Autodesk Fusion 360 part; units mm, degrees
(part 4 of 14)
  line L1260 (69.7278, -120.65) -> (64.2286, -111.125)
  line L1261 (64.2286, -130.175) -> (69.7278, -120.65)
  line L1262 (83.476, -100.0125) -> (72.4775, -100.0125)
  line L1263 (72.4775, -100.0125) -> (66.9782, -109.5375)
  line L1264 (66.9782, -109.5375) -> (72.4775, -119.0625)
  line L1265 (72.4775, -119.0625) -> (83.476, -119.0625)
  line L1266 (88.9753, -109.5375) -> (83.476, -100.0125)
  line L1267 (83.476, -119.0625) -> (88.9753, -109.5375)
  line L1268 (102.7234, -88.9) -> (91.7249, -88.9)
  line L1269 (91.7249, -88.9) -> (86.2256, -98.425)
  line L1270 (86.2256, -98.425) -> (91.7249, -107.95)
  line L1271 (91.7249, -107.95) -> (102.7234, -107.95)
  line L1272 (108.2227, -98.425) -> (102.7234, -88.9)
  line L1273 (102.7234, -107.95) -> (108.2227, -98.425)
  line L1274 (121.9708, -77.7875) -> (110.9723, -77.7875)
  line L1275 (110.9723, -77.7875) -> (105.473, -87.3125)
  line L1276 (105.473, -87.3125) -> (110.9723, -96.8375)
  line L1277 (110.9723, -96.8375) -> (121.9708, -96.8375)
  line L1278 (127.4701, -87.3125) -> (121.9708, -77.7875)
  line L1279 (121.9708, -96.8375) -> (127.4701, -87.3125)
  line L1280 (141.2182, -66.675) -> (130.2197, -66.675)
  line L1281 (130.2197, -66.675) -> (124.7205, -76.2)
  line L1282 (124.7205, -76.2) -> (130.2197, -85.725)
  line L1283 (130.2197, -85.725) -> (141.2182, -85.725)
  line L1284 (146.7175, -76.2) -> (141.2182, -66.675)
  line L1285 (141.2182, -85.725) -> (146.7175, -76.2)
  line L1286 (160.4657, -55.5625) -> (149.4671, -55.5625)
  line L1287 (149.4671, -55.5625) -> (143.9679, -65.0875)
  line L1288 (143.9679, -65.0875) -> (149.4671, -74.6125)
  line L1289 (149.4671, -74.6125) -> (160.4657, -74.6125)
  line L1290 (165.9649, -65.0875) -> (160.4657, -55.5625)
  line L1291 (160.4657, -74.6125) -> (165.9649, -65.0875)
  line L1292 (179.7131, -44.45) -> (168.7145, -44.45)
  line L1293 (168.7145, -44.45) -> (163.2153, -53.975)
  line L1294 (163.2153, -53.975) -> (168.7145, -63.5)
  line L1295 (168.7145, -63.5) -> (179.7131, -63.5)
  line L1296 (185.2123, -53.975) -> (179.7131, -44.45)
  line L1297 (179.7131, -63.5) -> (185.2123, -53.975)
  line L1298 (198.9605, -33.3375) -> (187.962, -33.3375)
  line L1299 (187.962, -33.3375) -> (182.4627, -42.8625)
  line L1300 (182.4627, -42.8625) -> (187.962, -52.3875)
  line L1301 (187.962, -52.3875) -> (198.9605, -52.3875)
  line L1302 (204.4597, -42.8625) -> (198.9605, -33.3375)
  line L1303 (198.9605, -52.3875) -> (204.4597, -42.8625)
  line L1304 (218.2079, -22.225) -> (207.2094, -22.225)
  line L1305 (207.2094, -22.225) -> (201.7101, -31.75)
  line L1306 (201.7101, -31.75) -> (207.2094, -41.275)
  line L1307 (207.2094, -41.275) -> (218.2079, -41.275)
  line L1308 (223.7072, -31.75) -> (218.2079, -22.225)
  line L1309 (218.2079, -41.275) -> (223.7072, -31.75)
  line L1310 (237.4553, -11.1125) -> (226.4568, -11.1125)
  line L1311 (226.4568, -11.1125) -> (220.9575, -20.6375)
  line L1312 (220.9575, -20.6375) -> (226.4568, -30.1625)
  line L1313 (226.4568, -30.1625) -> (237.4553, -30.1625)
  line L1314 (242.9546, -20.6375) -> (237.4553, -11.1125)
  line L1315 (237.4553, -30.1625) -> (242.9546, -20.6375)
  line L1316 (256.7027, 0) -> (245.7042, 0)
  line L1317 (245.7042, 0) -> (240.2049, -9.525)
  line L1318 (240.2049, -9.525) -> (245.7042, -19.05)
  line L1319 (245.7042, -19.05) -> (256.7027, -19.05)
  line L1320 (262.202, -9.525) -> (256.7027, 0)
  line L1321 (256.7027, -19.05) -> (262.202, -9.525)
  line L1322 (275.9501, 11.1125) -> (264.9516, 11.1125)
  line L1323 (264.9516, 11.1125) -> (259.4524, 1.5875)
  line L1324 (259.4524, 1.5875) -> (264.9516, -7.9375)
  line L1325 (264.9516, -7.9375) -> (275.9501, -7.9375)
  line L1326 (281.4494, 1.5875) -> (275.9501, 11.1125)
  line L1327 (275.9501, -7.9375) -> (281.4494, 1.5875)
  line L1328 (295.1976, 22.225) -> (284.199, 22.225)
  line L1329 (284.199, 22.225) -> (278.6998, 12.7)
  line L1330 (278.6998, 12.7) -> (284.199, 3.175)
  line L1331 (284.199, 3.175) -> (295.1976, 3.175)
  line L1332 (300.6968, 12.7) -> (295.1976, 22.225)
  line L1333 (295.1976, 3.175) -> (300.6968, 12.7)
  line L1334 (314.445, 33.3375) -> (303.4464, 33.3375)
  line L1335 (303.4464, 33.3375) -> (297.9472, 23.8125)
  line L1336 (297.9472, 23.8125) -> (303.4464, 14.2875)
  line L1337 (303.4464, 14.2875) -> (314.445, 14.2875)
  line L1338 (319.9442, 23.8125) -> (314.445, 33.3375)
  line L1339 (314.445, 14.2875) -> (319.9442, 23.8125)
  line L1340 (333.6924, 44.45) -> (322.6939, 44.45)
  line L1341 (322.6939, 44.45) -> (317.1946, 34.925)
  line L1342 (317.1946, 34.925) -> (322.6939, 25.4)
  line L1343 (322.6939, 25.4) -> (333.6924, 25.4)
  line L1344 (339.1916, 34.925) -> (333.6924, 44.45)
  line L1345 (333.6924, 25.4) -> (339.1916, 34.925)
  line L1346 (352.9398, 55.5625) -> (341.9413, 55.5625)
  line L1347 (341.9413, 55.5625) -> (336.442, 46.0375)
  line L1348 (336.442, 46.0375) -> (341.9413, 36.5125)
  line L1349 (341.9413, 36.5125) -> (352.9398, 36.5125)
  line L1350 (358.4391, 46.0375) -> (352.9398, 55.5625)
  line L1351 (352.9398, 36.5125) -> (358.4391, 46.0375)
  line L1352 (372.1872, 66.675) -> (361.1887, 66.675)
  line L1353 (361.1887, 66.675) -> (355.6894, 57.15)
  line L1354 (355.6894, 57.15) -> (361.1887, 47.625)
  line L1355 (361.1887, 47.625) -> (372.1872, 47.625)
  line L1356 (377.6865, 57.15) -> (372.1872, 66.675)
  line L1357 (372.1872, 47.625) -> (377.6865, 57.15)
  line L1358 (391.4346, 77.7875) -> (380.4361, 77.7875)
  line L1359 (380.4361, 77.7875) -> (374.9368, 68.2625)
  line L1360 (374.9368, 68.2625) -> (380.4361, 58.7375)
  line L1361 (380.4361, 58.7375) -> (391.4346, 58.7375)
  line L1362 (396.9339, 68.2625) -> (391.4346, 77.7875)
  line L1363 (391.4346, 58.7375) -> (396.9339, 68.2625)
  line L1364 (410.682, 88.9) -> (399.6835, 88.9)
  line L1365 (399.6835, 88.9) -> (394.1843, 79.375)
  line L1366 (394.1843, 79.375) -> (399.6835, 69.85)
  line L1367 (399.6835, 69.85) -> (410.682, 69.85)
  line L1368 (416.1813, 79.375) -> (410.682, 88.9)
  line L1369 (410.682, 69.85) -> (416.1813, 79.375)
  line L1370 (429.9295, 100.0125) -> (418.9309, 100.0125)
  line L1371 (418.9309, 100.0125) -> (413.4317, 90.4875)
  line L1372 (413.4317, 90.4875) -> (418.9309, 80.9625)
  line L1373 (418.9309, 80.9625) -> (429.9295, 80.9625)
  line L1374 (435.4287, 90.4875) -> (429.9295, 100.0125)
  line L1375 (429.9295, 80.9625) -> (435.4287, 90.4875)
  line L1376 (449.1769, 111.125) -> (438.1783, 111.125)
  line L1377 (438.1783, 111.125) -> (432.6791, 101.6)
  line L1378 (432.6791, 101.6) -> (438.1783, 92.075)
  line L1379 (438.1783, 92.075) -> (449.1769, 92.075)
  line L1380 (454.6761, 101.6) -> (449.1769, 111.125)
  line L1381 (449.1769, 92.075) -> (454.6761, 101.6)
  line L1382 (468.4243, 122.2375) -> (457.4258, 122.2375)
  line L1383 (457.4258, 122.2375) -> (451.9265, 112.7125)
  line L1384 (451.9265, 112.7125) -> (457.4258, 103.1875)
  line L1385 (457.4258, 103.1875) -> (468.4243, 103.1875)
  line L1386 (473.9235, 112.7125) -> (468.4243, 122.2375)
  line L1387 (468.4243, 103.1875) -> (473.9235, 112.7125)
  line L1388 (487.6717, 133.35) -> (476.6732, 133.35)
  line L1389 (476.6732, 133.35) -> (471.1739, 123.825)
  line L1390 (471.1739, 123.825) -> (476.6732, 114.3)
  line L1391 (476.6732, 114.3) -> (487.6717, 114.3)
  line L1392 (493.171, 123.825) -> (487.6717, 133.35)
  line L1393 (487.6717, 114.3) -> (493.171, 123.825)
  line L1394 (506.9191, 144.4625) -> (495.9206, 144.4625)
  line L1395 (495.9206, 144.4625) -> (490.4213, 134.9375)
  line L1396 (490.4213, 134.9375) -> (495.9206, 125.4125)
  line L1397 (495.9206, 125.4125) -> (506.9191, 125.4125)
  line L1398 (512.4184, 134.9375) -> (506.9191, 144.4625)
  line L1399 (506.9191, 125.4125) -> (512.4184, 134.9375)
  line L1400 (526.1665, 155.575) -> (515.168, 155.575)
  line L1401 (515.168, 155.575) -> (509.6687, 146.05)
  line L1402 (509.6687, 146.05) -> (515.168, 136.525)
  line L1403 (515.168, 136.525) -> (526.1665, 136.525)
  line L1404 (531.6658, 146.05) -> (526.1665, 155.575)
  line L1405 (526.1665, 136.525) -> (531.6658, 146.05)
  line L1406 (545.4139, 166.6875) -> (534.4154, 166.6875)
  line L1407 (534.4154, 166.6875) -> (528.9162, 157.1625)
  line L1408 (528.9162, 157.1625) -> (534.4154, 147.6375)
  line L1409 (534.4154, 147.6375) -> (545.4139, 147.6375)
  line L1410 (550.9132, 157.1625) -> (545.4139, 166.6875)
  line L1411 (545.4139, 147.6375) -> (550.9132, 157.1625)
  line L1412 (564.6614, 177.8) -> (553.6628, 177.8)
  line L1413 (553.6628, 177.8) -> (548.1636, 168.275)
  line L1414 (548.1636, 168.275) -> (553.6628, 158.75)
  line L1415 (553.6628, 158.75) -> (564.6614, 158.75)
  line L1416 (570.1606, 168.275) -> (564.6614, 177.8)
  line L1417 (564.6614, 158.75) -> (570.1606, 168.275)
  line L1418 (583.9088, 188.9125) -> (572.9102, 188.9125)
  line L1419 (572.9102, 188.9125) -> (567.411, 179.3875)
  line L1420 (567.411, 179.3875) -> (572.9102, 169.8625)
  line L1421 (572.9102, 169.8625) -> (583.9088, 169.8625)
  line L1422 (589.408, 179.3875) -> (583.9088, 188.9125)
  line L1423 (583.9088, 169.8625) -> (589.408, 179.3875)
  line L1424 (603.1562, 200.025) -> (592.1577, 200.025)
  line L1425 (592.1577, 200.025) -> (586.6584, 190.5)
  line L1426 (586.6584, 190.5) -> (592.1577, 180.975)
  line L1427 (592.1577, 180.975) -> (603.1562, 180.975)
  line L1428 (608.6554, 190.5) -> (603.1562, 200.025)
  line L1429 (603.1562, 180.975) -> (608.6554, 190.5)
  line L1430 (622.4036, 211.1375) -> (611.4051, 211.1375)
  line L1431 (611.4051, 211.1375) -> (605.9058, 201.6125)
  line L1432 (605.9058, 201.6125) -> (611.4051, 192.0875)
  line L1433 (611.4051, 192.0875) -> (622.4036, 192.0875)
  line L1434 (627.9029, 201.6125) -> (622.4036, 211.1375)
  line L1435 (622.4036, 192.0875) -> (627.9029, 201.6125)
  line L1436 (641.651, 222.25) -> (630.6525, 222.25)
  line L1437 (630.6525, 222.25) -> (625.1532, 212.725)
  line L1438 (625.1532, 212.725) -> (630.6525, 203.2)
  line L1439 (630.6525, 203.2) -> (641.651, 203.2)
  line L1440 (647.1503, 212.725) -> (641.651, 222.25)
  line L1441 (641.651, 203.2) -> (647.1503, 212.725)
  line L1442 (660.8984, 233.3625) -> (649.8999, 233.3625)
  line L1443 (649.8999, 233.3625) -> (644.4006, 223.8375)
  line L1444 (644.4006, 223.8375) -> (649.8999, 214.3125)
  line L1445 (649.8999, 214.3125) -> (660.8984, 214.3125)
  line L1446 (666.3977, 223.8375) -> (660.8984, 233.3625)
  line L1447 (660.8984, 214.3125) -> (666.3977, 223.8375)
  line L1448 (680.1458, 244.475) -> (669.1473, 244.475)
  line L1449 (669.1473, 244.475) -> (663.6481, 234.95)
  line L1450 (663.6481, 234.95) -> (669.1473, 225.425)
  line L1451 (669.1473, 225.425) -> (680.1458, 225.425)
  line L1452 (685.6451, 234.95) -> (680.1458, 244.475)
  line L1453 (680.1458, 225.425) -> (685.6451, 234.95)
  line L1454 (699.3933, 255.5875) -> (688.3947, 255.5875)
  line L1455 (688.3947, 255.5875) -> (682.8955, 246.0625)
  line L1456 (682.8955, 246.0625) -> (688.3947, 236.5375)
  line L1457 (688.3947, 236.5375) -> (699.3933, 236.5375)
  line L1458 (704.8925, 246.0625) -> (699.3933, 255.5875)
  line L1459 (699.3933, 236.5375) -> (704.8925, 246.0625)
  line L1460 (-455.4516, -388.9375) -> (-466.4501, -388.9375)
  line L1461 (-466.4501, -388.9375) -> (-471.9494, -398.4625)
  line L1462 (-471.9494, -398.4625) -> (-466.4501, -407.9875)
  line L1463 (-466.4501, -407.9875) -> (-455.4516, -407.9875)
  line L1464 (-449.9524, -398.4625) -> (-455.4516, -388.9375)
  line L1465 (-455.4516, -407.9875) -> (-449.9524, -398.4625)
  line L1466 (-436.2042, -377.825) -> (-447.2027, -377.825)
  line L1467 (-447.2027, -377.825) -> (-452.702, -387.35)
  line L1468 (-452.702, -387.35) -> (-447.2027, -396.875)
  line L1469 (-447.2027, -396.875) -> (-436.2042, -396.875)
  line L1470 (-430.7049, -387.35) -> (-436.2042, -377.825)
  line L1471 (-436.2042, -396.875) -> (-430.7049, -387.35)
  line L1472 (-416.9568, -366.7125) -> (-427.9553, -366.7125)
  line L1473 (-427.9553, -366.7125) -> (-433.4546, -376.2375)
  line L1474 (-433.4546, -376.2375) -> (-427.9553, -385.7625)
  line L1475 (-427.9553, -385.7625) -> (-416.9568, -385.7625)
  line L1476 (-411.4575, -376.2375) -> (-416.9568, -366.7125)
  line L1477 (-416.9568, -385.7625) -> (-411.4575, -376.2375)
  line L1478 (-397.7094, -355.6) -> (-408.7079, -355.6)
  line L1479 (-408.7079, -355.6) -> (-414.2072, -365.125)
  line L1480 (-414.2072, -365.125) -> (-408.7079, -374.65)
  line L1481 (-408.7079, -374.65) -> (-397.7094, -374.65)
  line L1482 (-392.2101, -365.125) -> (-397.7094, -355.6)
  line L1483 (-397.7094, -374.65) -> (-392.2101, -365.125)
  line L1484 (-378.462, -344.4875) -> (-389.4605, -344.4875)
  line L1485 (-389.4605, -344.4875) -> (-394.9597, -354.0125)
  line L1486 (-394.9597, -354.0125) -> (-389.4605, -363.5375)
  line L1487 (-389.4605, -363.5375) -> (-378.462, -363.5375)
  line L1488 (-372.9627, -354.0125) -> (-378.462, -344.4875)
  line L1489 (-378.462, -363.5375) -> (-372.9627, -354.0125)
  line L1490 (-359.2145, -333.375) -> (-370.2131, -333.375)
  line L1491 (-370.2131, -333.375) -> (-375.7123, -342.9)
  line L1492 (-375.7123, -342.9) -> (-370.2131, -352.425)
  line L1493 (-370.2131, -352.425) -> (-359.2145, -352.425)
  line L1494 (-353.7153, -342.9) -> (-359.2145, -333.375)
  line L1495 (-359.2145, -352.425) -> (-353.7153, -342.9)
  line L1496 (-339.9671, -322.2625) -> (-350.9657, -322.2625)
  line L1497 (-350.9657, -322.2625) -> (-356.4649, -331.7875)
  line L1498 (-356.4649, -331.7875) -> (-350.9657, -341.3125)
  line L1499 (-350.9657, -341.3125) -> (-339.9671, -341.3125)
  line L1500 (-334.4679, -331.7875) -> (-339.9671, -322.2625)
  line L1501 (-339.9671, -341.3125) -> (-334.4679, -331.7875)
  line L1502 (-320.7197, -311.15) -> (-331.7182, -311.15)
  line L1503 (-331.7182, -311.15) -> (-337.2175, -320.675)
  line L1504 (-337.2175, -320.675) -> (-331.7182, -330.2)
  line L1505 (-331.7182, -330.2) -> (-320.7197, -330.2)
  line L1506 (-315.2205, -320.675) -> (-320.7197, -311.15)
  line L1507 (-320.7197, -330.2) -> (-315.2205, -320.675)
  line L1508 (-301.4723, -300.0375) -> (-312.4708, -300.0375)
  line L1509 (-312.4708, -300.0375) -> (-317.9701, -309.5625)
  line L1510 (-317.9701, -309.5625) -> (-312.4708, -319.0875)
  line L1511 (-312.4708, -319.0875) -> (-301.4723, -319.0875)
  line L1512 (-295.973, -309.5625) -> (-301.4723, -300.0375)
  line L1513 (-301.4723, -319.0875) -> (-295.973, -309.5625)
  line L1514 (-282.2249, -288.925) -> (-293.2234, -288.925)
  line L1515 (-293.2234, -288.925) -> (-298.7227, -298.45)
  line L1516 (-298.7227, -298.45) -> (-293.2234, -307.975)
  line L1517 (-293.2234, -307.975) -> (-282.2249, -307.975)
  line L1518 (-276.7256, -298.45) -> (-282.2249, -288.925)
  line L1519 (-282.2249, -307.975) -> (-276.7256, -298.45)
  line L1520 (-262.9775, -277.8125) -> (-273.976, -277.8125)
  line L1521 (-273.976, -277.8125) -> (-279.4753, -287.3375)
  line L1522 (-279.4753, -287.3375) -> (-273.976, -296.8625)
  line L1523 (-273.976, -296.8625) -> (-262.9775, -296.8625)
  line L1524 (-257.4782, -287.3375) -> (-262.9775, -277.8125)
  line L1525 (-262.9775, -296.8625) -> (-257.4782, -287.3375)
  line L1526 (-243.7301, -266.7) -> (-254.7286, -266.7)
  line L1527 (-254.7286, -266.7) -> (-260.2278, -276.225)
  line L1528 (-260.2278, -276.225) -> (-254.7286, -285.75)
  line L1529 (-254.7286, -285.75) -> (-243.7301, -285.75)
  line L1530 (-238.2308, -276.225) -> (-243.7301, -266.7)
  line L1531 (-243.7301, -285.75) -> (-238.2308, -276.225)
  line L1532 (-224.4826, -255.5875) -> (-235.4812, -255.5875)
  line L1533 (-235.4812, -255.5875) -> (-240.9804, -265.1125)
  line L1534 (-240.9804, -265.1125) -> (-235.4812, -274.6375)
  line L1535 (-235.4812, -274.6375) -> (-224.4826, -274.6375)
  line L1536 (-218.9834, -265.1125) -> (-224.4826, -255.5875)
  line L1537 (-224.4826, -274.6375) -> (-218.9834, -265.1125)
  line L1538 (-205.2352, -244.475) -> (-216.2337, -244.475)
  line L1539 (-216.2337, -244.475) -> (-221.733, -254)
  line L1540 (-221.733, -254) -> (-216.2337, -263.525)
  line L1541 (-216.2337, -263.525) -> (-205.2352, -263.525)
  line L1542 (-199.736, -254) -> (-205.2352, -244.475)
  line L1543 (-205.2352, -263.525) -> (-199.736, -254)
  line L1544 (-185.9878, -233.3625) -> (-196.9863, -233.3625)
  line L1545 (-196.9863, -233.3625) -> (-202.4856, -242.8875)
  line L1546 (-202.4856, -242.8875) -> (-196.9863, -252.4125)
  line L1547 (-196.9863, -252.4125) -> (-185.9878, -252.4125)
  line L1548 (-180.4886, -242.8875) -> (-185.9878, -233.3625)
  line L1549 (-185.9878, -252.4125) -> (-180.4886, -242.8875)
  line L1550 (-166.7404, -222.25) -> (-177.7389, -222.25)
  line L1551 (-177.7389, -222.25) -> (-183.2382, -231.775)
  line L1552 (-183.2382, -231.775) -> (-177.7389, -241.3)
  line L1553 (-177.7389, -241.3) -> (-166.7404, -241.3)
  line L1554 (-161.2411, -231.775) -> (-166.7404, -222.25)
  line L1555 (-166.7404, -241.3) -> (-161.2411, -231.775)
  line L1556 (-147.493, -211.1375) -> (-158.4915, -211.1375)
  line L1557 (-158.4915, -211.1375) -> (-163.9908, -220.6625)
  line L1558 (-163.9908, -220.6625) -> (-158.4915, -230.1875)
  line L1559 (-158.4915, -230.1875) -> (-147.493, -230.1875)
  line L1560 (-141.9937, -220.6625) -> (-147.493, -211.1375)
  line L1561 (-147.493, -230.1875) -> (-141.9937, -220.6625)
  line L1562 (-128.2456, -200.025) -> (-139.2441, -200.025)
  line L1563 (-139.2441, -200.025) -> (-144.7434, -209.55)
  line L1564 (-144.7434, -209.55) -> (-139.2441, -219.075)
  line L1565 (-139.2441, -219.075) -> (-128.2456, -219.075)
  line L1566 (-122.7463, -209.55) -> (-128.2456, -200.025)
  line L1567 (-128.2456, -219.075) -> (-122.7463, -209.55)
  line L1568 (-108.9982, -188.9125) -> (-119.9967, -188.9125)
  line L1569 (-119.9967, -188.9125) -> (-125.4959, -198.4375)
  line L1570 (-125.4959, -198.4375) -> (-119.9967, -207.9625)
  line L1571 (-119.9967, -207.9625) -> (-108.9982, -207.9625)
  line L1572 (-103.4989, -198.4375) -> (-108.9982, -188.9125)
  line L1573 (-108.9982, -207.9625) -> (-103.4989, -198.4375)
  line L1574 (-89.7507, -177.8) -> (-100.7493, -177.8)
  line L1575 (-100.7493, -177.8) -> (-106.2485, -187.325)
  line L1576 (-106.2485, -187.325) -> (-100.7493, -196.85)
  line L1577 (-100.7493, -196.85) -> (-89.7507, -196.85)
  line L1578 (-84.2515, -187.325) -> (-89.7507, -177.8)
  line L1579 (-89.7507, -196.85) -> (-84.2515, -187.325)
  line L1580 (-70.5033, -166.6875) -> (-81.5018, -166.6875)
  line L1581 (-81.5018, -166.6875) -> (-87.0011, -176.2125)
  line L1582 (-87.0011, -176.2125) -> (-81.5018, -185.7375)
  line L1583 (-81.5018, -185.7375) -> (-70.5033, -185.7375)
  line L1584 (-65.0041, -176.2125) -> (-70.5033, -166.6875)
  line L1585 (-70.5033, -185.7375) -> (-65.0041, -176.2125)
  line L1586 (-51.2559, -155.575) -> (-62.2544, -155.575)
  line L1587 (-62.2544, -155.575) -> (-67.7537, -165.1)
  line L1588 (-67.7537, -165.1) -> (-62.2544, -174.625)
  line L1589 (-62.2544, -174.625) -> (-51.2559, -174.625)
  line L1590 (-45.7566, -165.1) -> (-51.2559, -155.575)
  line L1591 (-51.2559, -174.625) -> (-45.7566, -165.1)
  line L1592 (-32.0085, -144.4625) -> (-43.007, -144.4625)
  line L1593 (-43.007, -144.4625) -> (-48.5063, -153.9875)
  line L1594 (-48.5063, -153.9875) -> (-43.007, -163.5125)
  line L1595 (-43.007, -163.5125) -> (-32.0085, -163.5125)
  line L1596 (-26.5092, -153.9875) -> (-32.0085, -144.4625)
  line L1597 (-32.0085, -163.5125) -> (-26.5092, -153.9875)
  line L1598 (-12.7611, -133.35) -> (-23.7596, -133.35)
  line L1599 (-23.7596, -133.35) -> (-29.2589, -142.875)
  line L1600 (-29.2589, -142.875) -> (-23.7596, -152.4)
  line L1601 (-23.7596, -152.4) -> (-12.7611, -152.4)
  line L1602 (-7.2618, -142.875) -> (-12.7611, -133.35)
  line L1603 (-12.7611, -152.4) -> (-7.2618, -142.875)
  line L1604 (6.4863, -122.2375) -> (-4.5122, -122.2375)
  line L1605 (-4.5122, -122.2375) -> (-10.0114, -131.7625)
  line L1606 (-10.0114, -131.7625) -> (-4.5122, -141.2875)
  line L1607 (-4.5122, -141.2875) -> (6.4863, -141.2875)
  line L1608 (11.9856, -131.7625) -> (6.4863, -122.2375)
  line L1609 (6.4863, -141.2875) -> (11.9856, -131.7625)
  line L1610 (25.7337, -111.125) -> (14.7352, -111.125)
  line L1611 (14.7352, -111.125) -> (9.236, -120.65)
  line L1612 (9.236, -120.65) -> (14.7352, -130.175)
  line L1613 (14.7352, -130.175) -> (25.7337, -130.175)
  line L1614 (31.233, -120.65) -> (25.7337, -111.125)
  line L1615 (25.7337, -130.175) -> (31.233, -120.65)
  line L1616 (44.9812, -100.0125) -> (33.9826, -100.0125)
  line L1617 (33.9826, -100.0125) -> (28.4834, -109.5375)
  line L1618 (28.4834, -109.5375) -> (33.9826, -119.0625)
  line L1619 (33.9826, -119.0625) -> (44.9812, -119.0625)
  line L1620 (50.4804, -109.5375) -> (44.9812, -100.0125)
  line L1621 (44.9812, -119.0625) -> (50.4804, -109.5375)
  line L1622 (64.2286, -88.9) -> (53.2301, -88.9)
  line L1623 (53.2301, -88.9) -> (47.7308, -98.425)
  line L1624 (47.7308, -98.425) -> (53.2301, -107.95)
  line L1625 (53.2301, -107.95) -> (64.2286, -107.95)
  line L1626 (69.7278, -98.425) -> (64.2286, -88.9)
  line L1627 (64.2286, -107.95) -> (69.7278, -98.425)
  line L1628 (83.476, -77.7875) -> (72.4775, -77.7875)
  line L1629 (72.4775, -77.7875) -> (66.9782, -87.3125)
  line L1630 (66.9782, -87.3125) -> (72.4775, -96.8375)
  line L1631 (72.4775, -96.8375) -> (83.476, -96.8375)
  line L1632 (88.9753, -87.3125) -> (83.476, -77.7875)
  line L1633 (83.476, -96.8375) -> (88.9753, -87.3125)
  line L1634 (102.7234, -66.675) -> (91.7249, -66.675)
  line L1635 (91.7249, -66.675) -> (86.2256, -76.2)
  line L1636 (86.2256, -76.2) -> (91.7249, -85.725)
  line L1637 (91.7249, -85.725) -> (102.7234, -85.725)
  line L1638 (108.2227, -76.2) -> (102.7234, -66.675)
  line L1639 (102.7234, -85.725) -> (108.2227, -76.2)
  line L1640 (121.9708, -55.5625) -> (110.9723, -55.5625)
  line L1641 (110.9723, -55.5625) -> (105.473, -65.0875)
  line L1642 (105.473, -65.0875) -> (110.9723, -74.6125)
  line L1643 (110.9723, -74.6125) -> (121.9708, -74.6125)
  line L1644 (127.4701, -65.0875) -> (121.9708, -55.5625)
  line L1645 (121.9708, -74.6125) -> (127.4701, -65.0875)
  line L1646 (141.2182, -44.45) -> (130.2197, -44.45)
  line L1647 (130.2197, -44.45) -> (124.7205, -53.975)
  line L1648 (124.7205, -53.975) -> (130.2197, -63.5)
  line L1649 (130.2197, -63.5) -> (141.2182, -63.5)
  line L1650 (146.7175, -53.975) -> (141.2182, -44.45)
  line L1651 (141.2182, -63.5) -> (146.7175, -53.975)
  line L1652 (160.4657, -33.3375) -> (149.4671, -33.3375)
  line L1653 (149.4671, -33.3375) -> (143.9679, -42.8625)
  line L1654 (143.9679, -42.8625) -> (149.4671, -52.3875)
  line L1655 (149.4671, -52.3875) -> (160.4657, -52.3875)
  line L1656 (165.9649, -42.8625) -> (160.4657, -33.3375)
  line L1657 (160.4657, -52.3875) -> (165.9649, -42.8625)
  line L1658 (179.7131, -22.225) -> (168.7145, -22.225)
  line L1659 (168.7145, -22.225) -> (163.2153, -31.75)
  line L1660 (163.2153, -31.75) -> (168.7145, -41.275)
  line L1661 (168.7145, -41.275) -> (179.7131, -41.275)
  line L1662 (185.2123, -31.75) -> (179.7131, -22.225)
  line L1663 (179.7131, -41.275) -> (185.2123, -31.75)
  line L1664 (198.9605, -11.1125) -> (187.962, -11.1125)
  line L1665 (187.962, -11.1125) -> (182.4627, -20.6375)
  line L1666 (182.4627, -20.6375) -> (187.962, -30.1625)
  line L1667 (187.962, -30.1625) -> (198.9605, -30.1625)
  line L1668 (204.4597, -20.6375) -> (198.9605, -11.1125)
  line L1669 (198.9605, -30.1625) -> (204.4597, -20.6375)
  line L1670 (218.2079, 0) -> (207.2094, 0)
  line L1671 (207.2094, 0) -> (201.7101, -9.525)
  line L1672 (201.7101, -9.525) -> (207.2094, -19.05)
  line L1673 (207.2094, -19.05) -> (218.2079, -19.05)
  line L1674 (223.7072, -9.525) -> (218.2079, 0)
  line L1675 (218.2079, -19.05) -> (223.7072, -9.525)
  line L1676 (237.4553, 11.1125) -> (226.4568, 11.1125)
  line L1677 (226.4568, 11.1125) -> (220.9575, 1.5875)
  line L1678 (220.9575, 1.5875) -> (226.4568, -7.9375)
  line L1679 (226.4568, -7.9375) -> (237.4553, -7.9375)
  line L1680 (242.9546, 1.5875) -> (237.4553, 11.1125)
  line L1681 (237.4553, -7.9375) -> (242.9546, 1.5875)
  line L1682 (256.7027, 22.225) -> (245.7042, 22.225)
  line L1683 (245.7042, 22.225) -> (240.2049, 12.7)
  line L1684 (240.2049, 12.7) -> (245.7042, 3.175)
  line L1685 (245.7042, 3.175) -> (256.7027, 3.175)
  line L1686 (262.202, 12.7) -> (256.7027, 22.225)
  line L1687 (256.7027, 3.175) -> (262.202, 12.7)
  line L1688 (275.9501, 33.3375) -> (264.9516, 33.3375)
  line L1689 (264.9516, 33.3375) -> (259.4524, 23.8125)
  line L1690 (259.4524, 23.8125) -> (264.9516, 14.2875)
  line L1691 (264.9516, 14.2875) -> (275.9501, 14.2875)
  line L1692 (281.4494, 23.8125) -> (275.9501, 33.3375)
  line L1693 (275.9501, 14.2875) -> (281.4494, 23.8125)
  line L1694 (295.1976, 44.45) -> (284.199, 44.45)
  line L1695 (284.199, 44.45) -> (278.6998, 34.925)
  line L1696 (278.6998, 34.925) -> (284.199, 25.4)
  line L1697 (284.199, 25.4) -> (295.1976, 25.4)
  line L1698 (300.6968, 34.925) -> (295.1976, 44.45)
  line L1699 (295.1976, 25.4) -> (300.6968, 34.925)
  line L1700 (314.445, 55.5625) -> (303.4464, 55.5625)
  line L1701 (303.4464, 55.5625) -> (297.9472, 46.0375)
  line L1702 (297.9472, 46.0375) -> (303.4464, 36.5125)
  line L1703 (303.4464, 36.5125) -> (314.445, 36.5125)
  line L1704 (319.9442, 46.0375) -> (314.445, 55.5625)
  line L1705 (314.445, 36.5125) -> (319.9442, 46.0375)
  line L1706 (333.6924, 66.675) -> (322.6939, 66.675)
  line L1707 (322.6939, 66.675) -> (317.1946, 57.15)
  line L1708 (317.1946, 57.15) -> (322.6939, 47.625)
  line L1709 (322.6939, 47.625) -> (333.6924, 47.625)
  line L1710 (339.1916, 57.15) -> (333.6924, 66.675)
  line L1711 (333.6924, 47.625) -> (339.1916, 57.15)
  line L1712 (352.9398, 77.7875) -> (341.9413, 77.7875)
  line L1713 (341.9413, 77.7875) -> (336.442, 68.2625)
  line L1714 (336.442, 68.2625) -> (341.9413, 58.7375)
  line L1715 (341.9413, 58.7375) -> (352.9398, 58.7375)
  line L1716 (358.4391, 68.2625) -> (352.9398, 77.7875)
  line L1717 (352.9398, 58.7375) -> (358.4391, 68.2625)
  line L1718 (372.1872, 88.9) -> (361.1887, 88.9)
  line L1719 (361.1887, 88.9) -> (355.6894, 79.375)
  line L1720 (355.6894, 79.375) -> (361.1887, 69.85)
  line L1721 (361.1887, 69.85) -> (372.1872, 69.85)
  line L1722 (377.6865, 79.375) -> (372.1872, 88.9)
  line L1723 (372.1872, 69.85) -> (377.6865, 79.375)
  line L1724 (391.4346, 100.0125) -> (380.4361, 100.0125)
  line L1725 (380.4361, 100.0125) -> (374.9368, 90.4875)
  line L1726 (374.9368, 90.4875) -> (380.4361, 80.9625)
  line L1727 (380.4361, 80.9625) -> (391.4346, 80.9625)
  line L1728 (396.9339, 90.4875) -> (391.4346, 100.0125)
  line L1729 (391.4346, 80.9625) -> (396.9339, 90.4875)
  line L1730 (410.682, 111.125) -> (399.6835, 111.125)
  line L1731 (399.6835, 111.125) -> (394.1843, 101.6)
  line L1732 (394.1843, 101.6) -> (399.6835, 92.075)
  line L1733 (399.6835, 92.075) -> (410.682, 92.075)
  line L1734 (416.1813, 101.6) -> (410.682, 111.125)
  line L1735 (410.682, 92.075) -> (416.1813, 101.6)
  line L1736 (429.9295, 122.2375) -> (418.9309, 122.2375)
  line L1737 (418.9309, 122.2375) -> (413.4317, 112.7125)
  line L1738 (413.4317, 112.7125) -> (418.9309, 103.1875)
  line L1739 (418.9309, 103.1875) -> (429.9295, 103.1875)
  line L1740 (435.4287, 112.7125) -> (429.9295, 122.2375)
  line L1741 (429.9295, 103.1875) -> (435.4287, 112.7125)
  line L1742 (449.1769, 133.35) -> (438.1783, 133.35)
  line L1743 (438.1783, 133.35) -> (432.6791, 123.825)
  line L1744 (432.6791, 123.825) -> (438.1783, 114.3)
  line L1745 (438.1783, 114.3) -> (449.1769, 114.3)
  line L1746 (454.6761, 123.825) -> (449.1769, 133.35)
  line L1747 (449.1769, 114.3) -> (454.6761, 123.825)
  line L1748 (468.4243, 144.4625) -> (457.4258, 144.4625)
  line L1749 (457.4258, 144.4625) -> (451.9265, 134.9375)
  line L1750 (451.9265, 134.9375) -> (457.4258, 125.4125)
  line L1751 (457.4258, 125.4125) -> (468.4243, 125.4125)
  line L1752 (473.9235, 134.9375) -> (468.4243, 144.4625)
  line L1753 (468.4243, 125.4125) -> (473.9235, 134.9375)
  line L1754 (487.6717, 155.575) -> (476.6732, 155.575)
  line L1755 (476.6732, 155.575) -> (471.1739, 146.05)
  line L1756 (471.1739, 146.05) -> (476.6732, 136.525)
  line L1757 (476.6732, 136.525) -> (487.6717, 136.525)
  line L1758 (493.171, 146.05) -> (487.6717, 155.575)
  line L1759 (487.6717, 136.525) -> (493.171, 146.05)
  line L1760 (506.9191, 166.6875) -> (495.9206, 166.6875)
  line L1761 (495.9206, 166.6875) -> (490.4213, 157.1625)
  line L1762 (490.4213, 157.1625) -> (495.9206, 147.6375)
  line L1763 (495.9206, 147.6375) -> (506.9191, 147.6375)
  line L1764 (512.4184, 157.1625) -> (506.9191, 166.6875)
  line L1765 (506.9191, 147.6375) -> (512.4184, 157.1625)
  line L1766 (526.1665, 177.8) -> (515.168, 177.8)
  line L1767 (515.168, 177.8) -> (509.6687, 168.275)
  line L1768 (509.6687, 168.275) -> (515.168, 158.75)
  line L1769 (515.168, 158.75) -> (526.1665, 158.75)
  line L1770 (531.6658, 168.275) -> (526.1665, 177.8)
  line L1771 (526.1665, 158.75) -> (531.6658, 168.275)
  line L1772 (545.4139, 188.9125) -> (534.4154, 188.9125)
  line L1773 (534.4154, 188.9125) -> (528.9162, 179.3875)
  line L1774 (528.9162, 179.3875) -> (534.4154, 169.8625)
  line L1775 (534.4154, 169.8625) -> (545.4139, 169.8625)
  line L1776 (550.9132, 179.3875) -> (545.4139, 188.9125)
  line L1777 (545.4139, 169.8625) -> (550.9132, 179.3875)
  line L1778 (564.6614, 200.025) -> (553.6628, 200.025)
  line L1779 (553.6628, 200.025) -> (548.1636, 190.5)
  line L1780 (548.1636, 190.5) -> (553.6628, 180.975)
  line L1781 (553.6628, 180.975) -> (564.6614, 180.975)
  line L1782 (570.1606, 190.5) -> (564.6614, 200.025)
  line L1783 (564.6614, 180.975) -> (570.1606, 190.5)
  line L1784 (583.9088, 211.1375) -> (572.9102, 211.1375)
  line L1785 (572.9102, 211.1375) -> (567.411, 201.6125)
  line L1786 (567.411, 201.6125) -> (572.9102, 192.0875)
  line L1787 (572.9102, 192.0875) -> (583.9088, 192.0875)
  line L1788 (589.408, 201.6125) -> (583.9088, 211.1375)
  line L1789 (583.9088, 192.0875) -> (589.408, 201.6125)
  line L1790 (603.1562, 222.25) -> (592.1577, 222.25)
  line L1791 (592.1577, 222.25) -> (586.6584, 212.725)
  line L1792 (586.6584, 212.725) -> (592.1577, 203.2)
  line L1793 (592.1577, 203.2) -> (603.1562, 203.2)
  line L1794 (608.6554, 212.725) -> (603.1562, 222.25)
  line L1795 (603.1562, 203.2) -> (608.6554, 212.725)
  line L1796 (622.4036, 233.3625) -> (611.4051, 233.3625)
  line L1797 (611.4051, 233.3625) -> (605.9058, 223.8375)
  line L1798 (605.9058, 223.8375) -> (611.4051, 214.3125)
  line L1799 (611.4051, 214.3125) -> (622.4036, 214.3125)
  line L1800 (627.9029, 223.8375) -> (622.4036, 233.3625)
  line L1801 (622.4036, 214.3125) -> (627.9029, 223.8375)
  line L1802 (641.651, 244.475) -> (630.6525, 244.475)
  line L1803 (630.6525, 244.475) -> (625.1532, 234.95)
  line L1804 (625.1532, 234.95) -> (630.6525, 225.425)
  line L1805 (630.6525, 225.425) -> (641.651, 225.425)
  line L1806 (647.1503, 234.95) -> (641.651, 244.475)
  line L1807 (641.651, 225.425) -> (647.1503, 234.95)
  line L1808 (660.8984, 255.5875) -> (649.8999, 255.5875)
  line L1809 (649.8999, 255.5875) -> (644.4006, 246.0625)
  line L1810 (644.4006, 246.0625) -> (649.8999, 236.5375)
  line L1811 (649.8999, 236.5375) -> (660.8984, 236.5375)
  line L1812 (666.3977, 246.0625) -> (660.8984, 255.5875)
  line L1813 (660.8984, 236.5375) -> (666.3977, 246.0625)
  line L1814 (680.1458, 266.7) -> (669.1473, 266.7)
  line L1815 (669.1473, 266.7) -> (663.6481, 257.175)
  line L1816 (663.6481, 257.175) -> (669.1473, 247.65)
  line L1817 (669.1473, 247.65) -> (680.1458, 247.65)
  line L1818 (685.6451, 257.175) -> (680.1458, 266.7)
  line L1819 (680.1458, 247.65) -> (685.6451, 257.175)
  line L1820 (-474.699, -377.825) -> (-485.6976, -377.825)
  line L1821 (-485.6976, -377.825) -> (-491.1968, -387.35)
  line L1822 (-491.1968, -387.35) -> (-485.6976, -396.875)
  line L1823 (-485.6976, -396.875) -> (-474.699, -396.875)
  line L1824 (-469.1998, -387.35) -> (-474.699, -377.825)
  line L1825 (-474.699, -396.875) -> (-469.1998, -387.35)
  line L1826 (-455.4516, -366.7125) -> (-466.4501, -366.7125)
  line L1827 (-466.4501, -366.7125) -> (-471.9494, -376.2375)
  line L1828 (-471.9494, -376.2375) -> (-466.4501, -385.7625)
  line L1829 (-466.4501, -385.7625) -> (-455.4516, -385.7625)
  line L1830 (-449.9524, -376.2375) -> (-455.4516, -366.7125)
  line L1831 (-455.4516, -385.7625) -> (-449.9524, -376.2375)
  line L1832 (-436.2042, -355.6) -> (-447.2027, -355.6)
  line L1833 (-447.2027, -355.6) -> (-452.702, -365.125)
  line L1834 (-452.702, -365.125) -> (-447.2027, -374.65)
  line L1835 (-447.2027, -374.65) -> (-436.2042, -374.65)
  line L1836 (-430.7049, -365.125) -> (-436.2042, -355.6)
  line L1837 (-436.2042, -374.65) -> (-430.7049, -365.125)
  line L1838 (-416.9568, -344.4875) -> (-427.9553, -344.4875)
  line L1839 (-427.9553, -344.4875) -> (-433.4546, -354.0125)
  line L1840 (-433.4546, -354.0125) -> (-427.9553, -363.5375)
  line L1841 (-427.9553, -363.5375) -> (-416.9568, -363.5375)
  line L1842 (-411.4575, -354.0125) -> (-416.9568, -344.4875)
  line L1843 (-416.9568, -363.5375) -> (-411.4575, -354.0125)
  line L1844 (-397.7094, -333.375) -> (-408.7079, -333.375)
  line L1845 (-408.7079, -333.375) -> (-414.2072, -342.9)
  line L1846 (-414.2072, -342.9) -> (-408.7079, -352.425)
  line L1847 (-408.7079, -352.425) -> (-397.7094, -352.425)
  line L1848 (-392.2101, -342.9) -> (-397.7094, -333.375)
  line L1849 (-397.7094, -352.425) -> (-392.2101, -342.9)
  line L1850 (-378.462, -322.2625) -> (-389.4605, -322.2625)
  line L1851 (-389.4605, -322.2625) -> (-394.9597, -331.7875)
  line L1852 (-394.9597, -331.7875) -> (-389.4605, -341.3125)
  line L1853 (-389.4605, -341.3125) -> (-378.462, -341.3125)
  line L1854 (-372.9627, -331.7875) -> (-378.462, -322.2625)
  line L1855 (-378.462, -341.3125) -> (-372.9627, -331.7875)
  line L1856 (-359.2145, -311.15) -> (-370.2131, -311.15)
  line L1857 (-370.2131, -311.15) -> (-375.7123, -320.675)
  line L1858 (-375.7123, -320.675) -> (-370.2131, -330.2)
  line L1859 (-370.2131, -330.2) -> (-359.2145, -330.2)
  line L1860 (-353.7153, -320.675) -> (-359.2145, -311.15)
  line L1861 (-359.2145, -330.2) -> (-353.7153, -320.675)
  line L1862 (-339.9671, -300.0375) -> (-350.9657, -300.0375)
  line L1863 (-350.9657, -300.0375) -> (-356.4649, -309.5625)
  line L1864 (-356.4649, -309.5625) -> (-350.9657, -319.0875)
  line L1865 (-350.9657, -319.0875) -> (-339.9671, -319.0875)
  line L1866 (-334.4679, -309.5625) -> (-339.9671, -300.0375)
  line L1867 (-339.9671, -319.0875) -> (-334.4679, -309.5625)
  line L1868 (-320.7197, -288.925) -> (-331.7182, -288.925)
  line L1869 (-331.7182, -288.925) -> (-337.2175, -298.45)
  line L1870 (-337.2175, -298.45) -> (-331.7182, -307.975)
  line L1871 (-331.7182, -307.975) -> (-320.7197, -307.975)
  line L1872 (-315.2205, -298.45) -> (-320.7197, -288.925)
  line L1873 (-320.7197, -307.975) -> (-315.2205, -298.45)
  line L1874 (-301.4723, -277.8125) -> (-312.4708, -277.8125)
  line L1875 (-312.4708, -277.8125) -> (-317.9701, -287.3375)
  line L1876 (-317.9701, -287.3375) -> (-312.4708, -296.8625)
  line L1877 (-312.4708, -296.8625) -> (-301.4723, -296.8625)
  line L1878 (-295.973, -287.3375) -> (-301.4723, -277.8125)
  line L1879 (-301.4723, -296.8625) -> (-295.973, -287.3375)
  line L1880 (-282.2249, -266.7) -> (-293.2234, -266.7)
  line L1881 (-293.2234, -266.7) -> (-298.7227, -276.225)
  line L1882 (-298.7227, -276.225) -> (-293.2234, -285.75)
  line L1883 (-293.2234, -285.75) -> (-282.2249, -285.75)
  line L1884 (-276.7256, -276.225) -> (-282.2249, -266.7)
  line L1885 (-282.2249, -285.75) -> (-276.7256, -276.225)
  line L1886 (-262.9775, -255.5875) -> (-273.976, -255.5875)
  line L1887 (-273.976, -255.5875) -> (-279.4753, -265.1125)
  line L1888 (-279.4753, -265.1125) -> (-273.976, -274.6375)
  line L1889 (-273.976, -274.6375) -> (-262.9775, -274.6375)
  line L1890 (-257.4782, -265.1125) -> (-262.9775, -255.5875)
  line L1891 (-262.9775, -274.6375) -> (-257.4782, -265.1125)
  line L1892 (-243.7301, -244.475) -> (-254.7286, -244.475)
  line L1893 (-254.7286, -244.475) -> (-260.2278, -254)
  line L1894 (-260.2278, -254) -> (-254.7286, -263.525)
  line L1895 (-254.7286, -263.525) -> (-243.7301, -263.525)
  line L1896 (-238.2308, -254) -> (-243.7301, -244.475)
  line L1897 (-243.7301, -263.525) -> (-238.2308, -254)
  line L1898 (-224.4826, -233.3625) -> (-235.4812, -233.3625)
  line L1899 (-235.4812, -233.3625) -> (-240.9804, -242.8875)
  line L1900 (-240.9804, -242.8875) -> (-235.4812, -252.4125)
  line L1901 (-235.4812, -252.4125) -> (-224.4826, -252.4125)
  line L1902 (-218.9834, -242.8875) -> (-224.4826, -233.3625)
  line L1903 (-224.4826, -252.4125) -> (-218.9834, -242.8875)
  line L1904 (-205.2352, -222.25) -> (-216.2337, -222.25)
  line L1905 (-216.2337, -222.25) -> (-221.733, -231.775)
  line L1906 (-221.733, -231.775) -> (-216.2337, -241.3)
  line L1907 (-216.2337, -241.3) -> (-205.2352, -241.3)
  line L1908 (-199.736, -231.775) -> (-205.2352, -222.25)
  line L1909 (-205.2352, -241.3) -> (-199.736, -231.775)
  line L1910 (-185.9878, -211.1375) -> (-196.9863, -211.1375)
  line L1911 (-196.9863, -211.1375) -> (-202.4856, -220.6625)
  line L1912 (-202.4856, -220.6625) -> (-196.9863, -230.1875)
  line L1913 (-196.9863, -230.1875) -> (-185.9878, -230.1875)
  line L1914 (-180.4886, -220.6625) -> (-185.9878, -211.1375)
  line L1915 (-185.9878, -230.1875) -> (-180.4886, -220.6625)
  line L1916 (-166.7404, -200.025) -> (-177.7389, -200.025)
  line L1917 (-177.7389, -200.025) -> (-183.2382, -209.55)
  line L1918 (-183.2382, -209.55) -> (-177.7389, -219.075)
  line L1919 (-177.7389, -219.075) -> (-166.7404, -219.075)
  line L1920 (-161.2411, -209.55) -> (-166.7404, -200.025)
  line L1921 (-166.7404, -219.075) -> (-161.2411, -209.55)
  line L1922 (-147.493, -188.9125) -> (-158.4915, -188.9125)
  line L1923 (-158.4915, -188.9125) -> (-163.9908, -198.4375)
  line L1924 (-163.9908, -198.4375) -> (-158.4915, -207.9625)
  line L1925 (-158.4915, -207.9625) -> (-147.493, -207.9625)
  line L1926 (-141.9937, -198.4375) -> (-147.493, -188.9125)
  line L1927 (-147.493, -207.9625) -> (-141.9937, -198.4375)
  line L1928 (-128.2456, -177.8) -> (-139.2441, -177.8)
  line L1929 (-139.2441, -177.8) -> (-144.7434, -187.325)
  line L1930 (-144.7434, -187.325) -> (-139.2441, -196.85)
  line L1931 (-139.2441, -196.85) -> (-128.2456, -196.85)
  line L1932 (-122.7463, -187.325) -> (-128.2456, -177.8)
  line L1933 (-128.2456, -196.85) -> (-122.7463, -187.325)
  line L1934 (-108.9982, -166.6875) -> (-119.9967, -166.6875)
  line L1935 (-119.9967, -166.6875) -> (-125.4959, -176.2125)
  line L1936 (-125.4959, -176.2125) -> (-119.9967, -185.7375)
  line L1937 (-119.9967, -185.7375) -> (-108.9982, -185.7375)
  line L1938 (-103.4989, -176.2125) -> (-108.9982, -166.6875)
  line L1939 (-108.9982, -185.7375) -> (-103.4989, -176.2125)
  line L1940 (-89.7507, -155.575) -> (-100.7493, -155.575)
  line L1941 (-100.7493, -155.575) -> (-106.2485, -165.1)
  line L1942 (-106.2485, -165.1) -> (-100.7493, -174.625)
  line L1943 (-100.7493, -174.625) -> (-89.7507, -174.625)
  line L1944 (-84.2515, -165.1) -> (-89.7507, -155.575)
  line L1945 (-89.7507, -174.625) -> (-84.2515, -165.1)
  line L1946 (-70.5033, -144.4625) -> (-81.5018, -144.4625)
  line L1947 (-81.5018, -144.4625) -> (-87.0011, -153.9875)
  line L1948 (-87.0011, -153.9875) -> (-81.5018, -163.5125)
  line L1949 (-81.5018, -163.5125) -> (-70.5033, -163.5125)
  line L1950 (-65.0041, -153.9875) -> (-70.5033, -144.4625)
  line L1951 (-70.5033, -163.5125) -> (-65.0041, -153.9875)
  line L1952 (-51.2559, -133.35) -> (-62.2544, -133.35)
  line L1953 (-62.2544, -133.35) -> (-67.7537, -142.875)
  line L1954 (-67.7537, -142.875) -> (-62.2544, -152.4)
  line L1955 (-62.2544, -152.4) -> (-51.2559, -152.4)
  line L1956 (-45.7566, -142.875) -> (-51.2559, -133.35)
  line L1957 (-51.2559, -152.4) -> (-45.7566, -142.875)
  line L1958 (-32.0085, -122.2375) -> (-43.007, -122.2375)
  line L1959 (-43.007, -122.2375) -> (-48.5063, -131.7625)
  line L1960 (-48.5063, -131.7625) -> (-43.007, -141.2875)
  line L1961 (-43.007, -141.2875) -> (-32.0085, -141.2875)
  line L1962 (-26.5092, -131.7625) -> (-32.0085, -122.2375)
  line L1963 (-32.0085, -141.2875) -> (-26.5092, -131.7625)
  line L1964 (-12.7611, -111.125) -> (-23.7596, -111.125)
  line L1965 (-23.7596, -111.125) -> (-29.2589, -120.65)
  line L1966 (-29.2589, -120.65) -> (-23.7596, -130.175)
  line L1967 (-23.7596, -130.175) -> (-12.7611, -130.175)
  line L1968 (-7.2618, -120.65) -> (-12.7611, -111.125)
  line L1969 (-12.7611, -130.175) -> (-7.2618, -120.65)
  line L1970 (6.4863, -100.0125) -> (-4.5122, -100.0125)
  line L1971 (-4.5122, -100.0125) -> (-10.0114, -109.5375)
  line L1972 (-10.0114, -109.5375) -> (-4.5122, -119.0625)
  line L1973 (-4.5122, -119.0625) -> (6.4863, -119.0625)
  line L1974 (11.9856, -109.5375) -> (6.4863, -100.0125)
  line L1975 (6.4863, -119.0625) -> (11.9856, -109.5375)
  line L1976 (25.7337, -88.9) -> (14.7352, -88.9)
  line L1977 (14.7352, -88.9) -> (9.236, -98.425)
  line L1978 (9.236, -98.425) -> (14.7352, -107.95)
  line L1979 (14.7352, -107.95) -> (25.7337, -107.95)
  line L1980 (31.233, -98.425) -> (25.7337, -88.9)
  line L1981 (25.7337, -107.95) -> (31.233, -98.425)
  line L1982 (44.9812, -77.7875) -> (33.9826, -77.7875)
  line L1983 (33.9826, -77.7875) -> (28.4834, -87.3125)
  line L1984 (28.4834, -87.3125) -> (33.9826, -96.8375)
  line L1985 (33.9826, -96.8375) -> (44.9812, -96.8375)
  line L1986 (50.4804, -87.3125) -> (44.9812, -77.7875)
  line L1987 (44.9812, -96.8375) -> (50.4804, -87.3125)
  line L1988 (64.2286, -66.675) -> (53.2301, -66.675)
  line L1989 (53.2301, -66.675) -> (47.7308, -76.2)
  line L1990 (47.7308, -76.2) -> (53.2301, -85.725)
  line L1991 (53.2301, -85.725) -> (64.2286, -85.725)
  line L1992 (69.7278, -76.2) -> (64.2286, -66.675)
  line L1993 (64.2286, -85.725) -> (69.7278, -76.2)
  line L1994 (83.476, -55.5625) -> (72.4775, -55.5625)
  line L1995 (72.4775, -55.5625) -> (66.9782, -65.0875)
  line L1996 (66.9782, -65.0875) -> (72.4775, -74.6125)
  line L1997 (72.4775, -74.6125) -> (83.476, -74.6125)
  line L1998 (88.9753, -65.0875) -> (83.476, -55.5625)
  line L1999 (83.476, -74.6125) -> (88.9753, -65.0875)
  line L2000 (102.7234, -44.45) -> (91.7249, -44.45)
  line L2001 (91.7249, -44.45) -> (86.2256, -53.975)
  line L2002 (86.2256, -53.975) -> (91.7249, -63.5)
  line L2003 (91.7249, -63.5) -> (102.7234, -63.5)
  line L2004 (108.2227, -53.975) -> (102.7234, -44.45)
  line L2005 (102.7234, -63.5) -> (108.2227, -53.975)
  line L2006 (121.9708, -33.3375) -> (110.9723, -33.3375)
  line L2007 (110.9723, -33.3375) -> (105.473, -42.8625)
  line L2008 (105.473, -42.8625) -> (110.9723, -52.3875)
  line L2009 (110.9723, -52.3875) -> (121.9708, -52.3875)
  line L2010 (127.4701, -42.8625) -> (121.9708, -33.3375)
  line L2011 (121.9708, -52.3875) -> (127.4701, -42.8625)
  line L2012 (141.2182, -22.225) -> (130.2197, -22.225)
  line L2013 (130.2197, -22.225) -> (124.7205, -31.75)
  line L2014 (124.7205, -31.75) -> (130.2197, -41.275)
  line L2015 (130.2197, -41.275) -> (141.2182, -41.275)
  line L2016 (146.7175, -31.75) -> (141.2182, -22.225)
  line L2017 (141.2182, -41.275) -> (146.7175, -31.75)
  line L2018 (160.4657, -11.1125) -> (149.4671, -11.1125)
  line L2019 (149.4671, -11.1125) -> (143.9679, -20.6375)
  line L2020 (143.9679, -20.6375) -> (149.4671, -30.1625)
  line L2021 (149.4671, -30.1625) -> (160.4657, -30.1625)
  line L2022 (165.9649, -20.6375) -> (160.4657, -11.1125)
  line L2023 (160.4657, -30.1625) -> (165.9649, -20.6375)
  line L2024 (179.7131, 0) -> (168.7145, 0)
  line L2025 (168.7145, 0) -> (163.2153, -9.525)
  line L2026 (163.2153, -9.525) -> (168.7145, -19.05)
  line L2027 (168.7145, -19.05) -> (179.7131, -19.05)
  line L2028 (185.2123, -9.525) -> (179.7131, 0)
  line L2029 (179.7131, -19.05) -> (185.2123, -9.525)
  line L2030 (198.9605, 11.1125) -> (187.962, 11.1125)
  line L2031 (187.962, 11.1125) -> (182.4627, 1.5875)
  line L2032 (182.4627, 1.5875) -> (187.962, -7.9375)
  line L2033 (187.962, -7.9375) -> (198.9605, -7.9375)
  line L2034 (204.4597, 1.5875) -> (198.9605, 11.1125)
  line L2035 (198.9605, -7.9375) -> (204.4597, 1.5875)
  line L2036 (218.2079, 22.225) -> (207.2094, 22.225)
  line L2037 (207.2094, 22.225) -> (201.7101, 12.7)
  line L2038 (201.7101, 12.7) -> (207.2094, 3.175)
  line L2039 (207.2094, 3.175) -> (218.2079, 3.175)
  line L2040 (223.7072, 12.7) -> (218.2079, 22.225)
  line L2041 (218.2079, 3.175) -> (223.7072, 12.7)
  line L2042 (237.4553, 33.3375) -> (226.4568, 33.3375)
  line L2043 (226.4568, 33.3375) -> (220.9575, 23.8125)
  line L2044 (220.9575, 23.8125) -> (226.4568, 14.2875)
  line L2045 (226.4568, 14.2875) -> (237.4553, 14.2875)
  line L2046 (242.9546, 23.8125) -> (237.4553, 33.3375)
  line L2047 (237.4553, 14.2875) -> (242.9546, 23.8125)
  line L2048 (256.7027, 44.45) -> (245.7042, 44.45)
  line L2049 (245.7042, 44.45) -> (240.2049, 34.925)
  line L2050 (240.2049, 34.925) -> (245.7042, 25.4)
  line L2051 (245.7042, 25.4) -> (256.7027, 25.4)
  line L2052 (262.202, 34.925) -> (256.7027, 44.45)
  line L2053 (256.7027, 25.4) -> (262.202, 34.925)
  line L2054 (275.9501, 55.5625) -> (264.9516, 55.5625)
  line L2055 (264.9516, 55.5625) -> (259.4524, 46.0375)
  line L2056 (259.4524, 46.0375) -> (264.9516, 36.5125)
  line L2057 (264.9516, 36.5125) -> (275.9501, 36.5125)
  line L2058 (281.4494, 46.0375) -> (275.9501, 55.5625)
  line L2059 (275.9501, 36.5125) -> (281.4494, 46.0375)
  line L2060 (295.1976, 66.675) -> (284.199, 66.675)
  line L2061 (284.199, 66.675) -> (278.6998, 57.15)
  line L2062 (278.6998, 57.15) -> (284.199, 47.625)
  line L2063 (284.199, 47.625) -> (295.1976, 47.625)
  line L2064 (300.6968, 57.15) -> (295.1976, 66.675)
  line L2065 (295.1976, 47.625) -> (300.6968, 57.15)
  line L2066 (314.445, 77.7875) -> (303.4464, 77.7875)
  line L2067 (303.4464, 77.7875) -> (297.9472, 68.2625)
  line L2068 (297.9472, 68.2625) -> (303.4464, 58.7375)
  line L2069 (303.4464, 58.7375) -> (314.445, 58.7375)
  line L2070 (319.9442, 68.2625) -> (314.445, 77.7875)
  line L2071 (314.445, 58.7375) -> (319.9442, 68.2625)
  line L2072 (333.6924, 88.9) -> (322.6939, 88.9)
  line L2073 (322.6939, 88.9) -> (317.1946, 79.375)
  line L2074 (317.1946, 79.375) -> (322.6939, 69.85)
  line L2075 (322.6939, 69.85) -> (333.6924, 69.85)
  line L2076 (339.1916, 79.375) -> (333.6924, 88.9)
  line L2077 (333.6924, 69.85) -> (339.1916, 79.375)
  line L2078 (352.9398, 100.0125) -> (341.9413, 100.0125)
  line L2079 (341.9413, 100.0125) -> (336.442, 90.4875)
  line L2080 (336.442, 90.4875) -> (341.9413, 80.9625)
  line L2081 (341.9413, 80.9625) -> (352.9398, 80.9625)
  line L2082 (358.4391, 90.4875) -> (352.9398, 100.0125)
  line L2083 (352.9398, 80.9625) -> (358.4391, 90.4875)
  line L2084 (372.1872, 111.125) -> (361.1887, 111.125)
  line L2085 (361.1887, 111.125) -> (355.6894, 101.6)
  line L2086 (355.6894, 101.6) -> (361.1887, 92.075)
  line L2087 (361.1887, 92.075) -> (372.1872, 92.075)
  line L2088 (377.6865, 101.6) -> (372.1872, 111.125)
  line L2089 (372.1872, 92.075) -> (377.6865, 101.6)
  line L2090 (391.4346, 122.2375) -> (380.4361, 122.2375)
  line L2091 (380.4361, 122.2375) -> (374.9368, 112.7125)
  line L2092 (374.9368, 112.7125) -> (380.4361, 103.1875)
  line L2093 (380.4361, 103.1875) -> (391.4346, 103.1875)
  line L2094 (396.9339, 112.7125) -> (391.4346, 122.2375)
  line L2095 (391.4346, 103.1875) -> (396.9339, 112.7125)
  line L2096 (410.682, 133.35) -> (399.6835, 133.35)
  line L2097 (399.6835, 133.35) -> (394.1843, 123.825)
  line L2098 (394.1843, 123.825) -> (399.6835, 114.3)
  line L2099 (399.6835, 114.3) -> (410.682, 114.3)
  line L2100 (416.1813, 123.825) -> (410.682, 133.35)
  line L2101 (410.682, 114.3) -> (416.1813, 123.825)
  line L2102 (429.9295, 144.4625) -> (418.9309, 144.4625)
  line L2103 (418.9309, 144.4625) -> (413.4317, 134.9375)
  line L2104 (413.4317, 134.9375) -> (418.9309, 125.4125)
  line L2105 (418.9309, 125.4125) -> (429.9295, 125.4125)
  line L2106 (435.4287, 134.9375) -> (429.9295, 144.4625)
  line L2107 (429.9295, 125.4125) -> (435.4287, 134.9375)
  line L2108 (449.1769, 155.575) -> (438.1783, 155.575)
  line L2109 (438.1783, 155.575) -> (432.6791, 146.05)
  line L2110 (432.6791, 146.05) -> (438.1783, 136.525)
  line L2111 (438.1783, 136.525) -> (449.1769, 136.525)
  line L2112 (454.6761, 146.05) -> (449.1769, 155.575)
  line L2113 (449.1769, 136.525) -> (454.6761, 146.05)
  line L2114 (468.4243, 166.6875) -> (457.4258, 166.6875)
  line L2115 (457.4258, 166.6875) -> (451.9265, 157.1625)
  line L2116 (451.9265, 157.1625) -> (457.4258, 147.6375)
  line L2117 (457.4258, 147.6375) -> (468.4243, 147.6375)
  line L2118 (473.9235, 157.1625) -> (468.4243, 166.6875)
  line L2119 (468.4243, 147.6375) -> (473.9235, 157.1625)
  line L2120 (487.6717, 177.8) -> (476.6732, 177.8)
  line L2121 (476.6732, 177.8) -> (471.1739, 168.275)
  line L2122 (471.1739, 168.275) -> (476.6732, 158.75)
  line L2123 (476.6732, 158.75) -> (487.6717, 158.75)
  line L2124 (493.171, 168.275) -> (487.6717, 177.8)
  line L2125 (487.6717, 158.75) -> (493.171, 168.275)
  line L2126 (506.9191, 188.9125) -> (495.9206, 188.9125)
  line L2127 (495.9206, 188.9125) -> (490.4213, 179.3875)
  line L2128 (490.4213, 179.3875) -> (495.9206, 169.8625)
  line L2129 (495.9206, 169.8625) -> (506.9191, 169.8625)
  line L2130 (512.4184, 179.3875) -> (506.9191, 188.9125)
  line L2131 (506.9191, 169.8625) -> (512.4184, 179.3875)
  line L2132 (526.1665, 200.025) -> (515.168, 200.025)
  line L2133 (515.168, 200.025) -> (509.6687, 190.5)
  line L2134 (509.6687, 190.5) -> (515.168, 180.975)
  line L2135 (515.168, 180.975) -> (526.1665, 180.975)
  line L2136 (531.6658, 190.5) -> (526.1665, 200.025)
  line L2137 (526.1665, 180.975) -> (531.6658, 190.5)
  line L2138 (545.4139, 211.1375) -> (534.4154, 211.1375)
  line L2139 (534.4154, 211.1375) -> (528.9162, 201.6125)